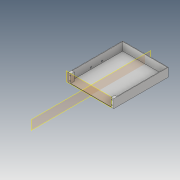
# Autodesk Inventor part: Case Tastiera
Saved by Autodesk Inventor 2019 (Build 230136000, 136)
## iProperties
Created: 2020-09-15
Part Number: Case Tastiera
Material: Generic
Document SubType Name: Modeling
Designer: giacomo
Density: 1 g/cm^3
Appearance: Default
Author: giacomo
Autodesk Inventor part; units mm, degrees
ref_plane "YZ Plane" through (0, 0, 0) normal (1, 0, 0) x (0, 1, 0)
ref_plane "XZ Plane" through (0, 0, 0) normal (0, 1, 0) x (-1, 0, 0)
ref_plane "XY Plane" through (0, 0, 0) normal (0, 0, 1) x (1, 0, 0)
sketch "Sketch1" plane through (0, 0, 0) normal (0, 1, 0) x (-1, 0, 0)
  line L0 (80.1493, 105.9266) -> (-24.8507, 105.9266) construction
  line L1 (-24.8507, 105.9266) -> (-24.8507, -189.0734) construction
  line L2 (-24.8507, -189.0734) -> (80.1493, -189.0734) construction
  line L3 (80.1493, -189.0734) -> (80.1493, 105.9266) construction
  line L4 (80.1493, 91.9266) -> (83.1493, 91.9266) construction
  line L5 (83.1493, 91.9266) -> (83.1493, 84.3266) construction
  line L6 (83.1493, 84.3266) -> (80.1493, 84.3266) construction
  line L7 (80.1493, 84.3266) -> (80.1493, 91.9266) construction
  point P0 (0, 0)
  dimension "d0" = 295
  dimension "d1" = 105
  dimension "d2" = 7.6
  dimension "d3" = 3
  dimension "d4" = 14
  constraints: 16 end point, 4 parallel, 2 horizontal, 2 perpendicular, 1 point on line
  measures "d0" distance of L2.end L0.start
  measures "d1" distance of L1.end L2.end
  measures "d2" distance of L4.end L5.end
  measures "d3" distance of L5.end L6.end
  measures "d4" distance between parallel lines of L0 L4
sketch "Sketch2" plane through (0, 0, 0) normal (0, 1, 0) x (-1, 0, 0)
  line L0 (80.1493, -189.0734) -> (80.1493, 105.9266) construction
  line L1 (-24.8507, -189.0734) -> (80.1493, -189.0734) construction
  line L2 (-24.8507, 105.9266) -> (-24.8507, -189.0734) construction
  line L3 (80.1493, 105.9266) -> (-24.8507, 105.9266) construction
  line L4 (90.1493, 109.9266) -> (90.1493, -193.0734)
  line L5 (-34.8507, -193.0734) -> (-34.8507, 109.9266)
  line L6 (90.1493, 109.9266) -> (-34.8507, 109.9266)
  line L7 (90.1493, -193.0734) -> (-34.8507, -193.0734)
  line L8 (91.6493, -194.5734) -> (91.6493, 111.4266)
  line L9 (91.6493, 111.4266) -> (-36.3507, 111.4266)
  line L10 (-36.3507, 111.4266) -> (-36.3507, -194.5734)
  line L11 (-36.3507, -194.5734) -> (91.6493, -194.5734)
  dimension "d71" = 10
  dimension "d72" = 4
  dimension "d73" = 10
  dimension "d74" = 4
  dimension "d75" = 1.5
  constraints: 16 end point, 2 parallel, 2 perpendicular, 3 other
  measures "d71" distance between parallel lines of L0 L4
  measures "d72" distance between parallel lines of L6 L3
  measures "d73" distance between parallel lines of L2 L5
  measures "d74" distance between parallel lines of L1 L7
  measures "d75" distance between parallel lines of L4 L8
extrude "Extrusion1" add sketch "Sketch2" against normal blind 1 contours L4 L7 L5 L6
extrude "Extrusion2" add sketch "Sketch2" along normal blind 23 and the other way blind 1
sketch "Sketch5" plane through (-91.6493, -1, 111.4266) normal (-1, 0, 0) x (0, 0, 1)
  circle A0 centre (-246, 6) radius 2.25
  circle A1 centre (-90.8, 6) radius 2.25
  circle A2 centre (-215.2, 6) radius 2.25
  circle A3 centre (-60, 6) radius 2.25
  line L0 (0, 0) -> (0, 24) projected
  line L1 (-306, 24) -> (0, 24) projected
  line L2 (-306, 24) -> (-306, 0) projected
  line L3 (0, 0) -> (-306, 0) projected
  point P0 (-111.4266, 1)
  dimension "d35" = 4.5
  dimension "d37" = 4.5
  dimension "d39" = 4.5
  dimension "d40" = 0
  dimension "d41" = 30.8
  dimension "d45" = 4.5
  dimension "d46" = 0
  dimension "d47" = 30.8
  dimension "d76" = 60
  dimension "d77" = 60
  dimension "d144" = 18
  dimension "d145" = 18
  constraints: 4 centre point
  measures "d35" diameter of A0
  measures "d37" diameter of A1
  measures "d39" diameter of A2
  measures "d40" vertical distance of A2.centre A0.centre
  measures "d41" distance of A2.centre A0.centre
  measures "d45" diameter of A3
  measures "d46" vertical distance of A3.centre A1.centre
  measures "d47" distance of A3.centre A1.centre
  measures "d76" distance from line of L2 A0.centre
  measures "d77" distance from line of L0 A3.centre
  measures "d144" distance from line of L1 A2.centre
  measures "d145" distance from line of L1 A1.centre
extrude "Extrusion4" cut sketch "Sketch5" against normal up to surface (1.5 mm away) contours A0 | A1 | A2 | A3
sketch "Sketch7" plane through (-90.1493, 0, -193.0734) normal (1, 0, 0) x (0, 0, -1)
  line L0 (-151.5, 23) -> (-151.5, 0) construction
  line L1 (-141.5, 23) -> (-141.5, 0)
  line L2 (-161.5, 23) -> (-161.5, 0)
  line L3 (-303, 23) -> (0, 23) projected
  line L4 (-303, 0) -> (0, 0) projected
  line L5 (0, 23) -> (0, 0) projected
  dimension "d106" = 10
  dimension "d107" = 10
  dimension "d148" = 151.5
  dimension "d149" = 151.5
  constraints: 6 end point
  measures "d106" distance between parallel lines of L1 L0
  measures "d107" distance between parallel lines of L2 L0
  measures "d148" distance from line of L3.start L0
  measures "d149" distance between parallel lines of L5 L0
extrude "Extrusion6" add sketch "Sketch7" along normal blind 6 contours L1 L4 L2 L3
ref_plane "Work Plane2" through (-27.6493, 0, 109.9266) normal (1, 0, 0) x (0, 0, -1)
ref_plane "Work Plane4" through (-90.1493, 0, -41.5734) normal (0, 0, 1) x (1, 0, 0)
sketch "Sketch16" plane through (-90.1493, 0, -31.5734) normal (0, 0, 1) x (1, 0, 0)
  line L0 (0, 0) -> (0, 23) projected
  line L1 (0, 23) -> (6, 23) projected
  point P0 (90.1493, 0)
  point P1 (3.5, 18)
  dimension "d108" = 3.5
  dimension "d109" = 5
  measures "d108" distance from line of L0 point (3.5, 18)
  measures "d109" distance from line of L1 point (3.5, 18)
hole "Hole3" at (-86.6493, 18, -31.5734) direction (0, 0, -1) diameter 2.6 depth 5 countersink diameter 5 countersink angle 82
sketch "Sketch17" plane through (-86.6493, 18, -36.5734) normal (0, 0, 1) x (1, 0, 0)
  circle A0 centre (0, 0) radius 1.3 projected
  point P0 (86.6493, -18)
  constraints: 1 coincident
hole "Hole4" at (-86.6493, 18, -36.5734) direction (0, 0, -1) diameter 2.6 depth 15 tip angle 118
sketch "Sketch18" plane through (-90.1493, 0, -31.5734) normal (0, 0, 1) x (1, 0, 0)
  line L0 (0, 0) -> (0, 23) projected
  line L1 (6, 0) -> (0, 0) projected
  point P0 (90.1493, 0)
  point P1 (3.5, 5)
  point P2 (0, 18)
  dimension "d124" = 3.5
  dimension "d125" = 5
  measures "d124" distance from line of L0 point (3.5, 5)
  measures "d125" distance from line of L1 point (3.5, 5)
hole "Hole5" at (-86.6493, 5, -31.5734) direction (0, 0, -1) diameter 2.6 depth 5 countersink diameter 5 countersink angle 82
sketch "Sketch19" plane through (-86.6493, 5, -36.5734) normal (0, 0, 1) x (1, 0, 0)
  circle A0 centre (0, 0) radius 1.3 projected
  point P0 (86.6493, -5)
  constraints: 1 coincident
hole "Hole6" at (-86.6493, 5, -36.5734) direction (0, 0, -1) diameter 2.6 depth 15 tip angle 118
mirror "Mirror6" about plane through (-27.6493, 0, 109.9266) normal (1, 0, 0) of "Extrusion6", "Hole3", "Hole5", "Hole4", "Hole6"
sketch "Sketch21" plane through (-90.1493, 0, -41.5734) normal (0, 0, 1) x (1, 0, 0)
  line L0 (-38.4696, 48.4578) -> (185.798, 48.4578)
  line L1 (185.798, 48.4578) -> (185.798, -48.9918)
  line L2 (185.798, -48.9918) -> (-38.4696, -48.9918)
  line L3 (-38.4696, -48.9918) -> (-38.4696, 48.4578)
  point P0 (90.1493, 0)
  constraints: 8 end point, 2 parallel, 1 horizontal, 1 perpendicular
extrude "Extrusion12" cut sketch "Sketch21" along normal through all
body "Solid1"
